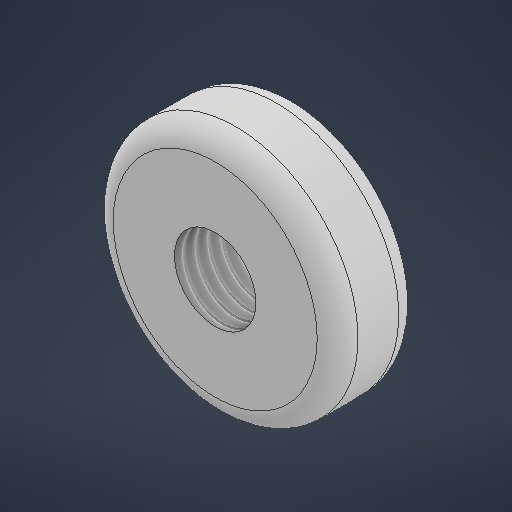
# Autodesk Inventor part: solar panel brush wheel
Saved by Autodesk Inventor 2026 (Build 300175050, 175E)
## iProperties
Created: 2026-02-12
Part Number: solar panel brush wheel
Material: Generic
Document SubType Name: Modeling
Designer: 268359
Density: 1 g/cm^3
Appearance: Default
Author: 268359
Autodesk Inventor part; units mm, degrees
ref_plane "YZ Plane" through (0, 0, 0) normal (1, 0, 0) x (0, 1, 0)
ref_plane "XZ Plane" through (0, 0, 0) normal (0, 1, 0) x (-1, 0, 0)
ref_plane "XY Plane" through (0, 0, 0) normal (0, 0, 1) x (1, 0, 0)
sketch "Sketch1" plane through (0, 0, 0) normal (0, 0, 1) x (1, 0, 0)
  arc A0 (19.05, 0) -> (-19.05, 0) centre (0, 0) ccw
  arc A1 (6.35, 0) -> (-6.35, 0) centre (0, 0) ccw
  line L0 (-19.05, 0) -> (-6.35, 0)
  line L1 (6.35, 0) -> (19.05, 0)
  arc A2 (-6.35, 0) -> (6.35, 0) centre (0, 0) ccw
  arc A3 (-19.05, 0) -> (19.05, 0) centre (0, 0) ccw
  point P0 (-6.35, 0)
  constraints: 8 point on circle, 4 centre point, 4 end point, 2 coincident, 2 concentric, 1 collinear, 1 horizontal
extrude "Extrusion1" add sketch "Sketch1" along normal blind 12.7 contours L1 A1 L0 A0 | A3 L0 A2 L1
fillet "Fillet1" radius 3.175 2 edges at (0, 19.05, 12.7) (0, 19.05, 0)
thread "Thread1" size "1/2-13 UNC" class "2B" standard "ANSI Unified Screw Threads" length 12.7
body "Solid1"
